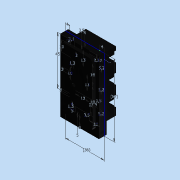
# Autodesk Inventor part: Base_V3
Saved by Autodesk Inventor 2015 (Build 190159000, 159)
## iProperties
Created: 2015-01-28
Part Number: Base_V3
Material: Generic
Document SubType Name: Modeling
Designer: Openlab
Density: 1 g/cm^3
Appearance: Smooth - Black
Author: Openlab
Autodesk Inventor part; units mm, degrees
ref_plane "YZ Plane" through (0, 0, 0) normal (1, 0, 0) x (0, 1, 0)
ref_plane "XZ Plane" through (0, 0, 0) normal (0, 1, 0) x (-1, 0, 0)
ref_plane "XY Plane" through (0, 0, 0) normal (0, 0, 1) x (1, 0, 0)
sketch "Sketch1" plane through (0, 0, 0) normal (0, 1, 0) x (-1, 0, 0)
  line L0 (23, -7.5) -> (10, -7.5)
  line L1 (10, -7.5) -> (10, -20.5)
  line L2 (10, -20.5) -> (23, -20.5)
  line L3 (10, -43.5) -> (10, -56.5)
  line L4 (10, -56.5) -> (23, -56.5)
  line L5 (23, -43.5) -> (10, -43.5)
  line L6 (0, -60) -> (0, 0)
  line L7 (28, -60) -> (0, -60)
  line L8 (23, -51.5) -> (28, -51.5)
  line L9 (28, -48.5) -> (23, -48.5)
  line L10 (24.85, -37) -> (26.15, -37)
  line L11 (26.15, -27) -> (24.85, -27)
  line L12 (28, -33.5) -> (26.15, -33.5)
  line L13 (24.85, -33.5) -> (23, -33.5)
  line L14 (28, -30.5) -> (26.15, -30.5)
  line L15 (24.85, -30.5) -> (23, -30.5)
  line L16 (23.95, -19) -> (27.05, -19)
  line L17 (27.05, -9) -> (23.95, -9)
  line L18 (23, -15.5) -> (23.95, -15.5)
  line L19 (27.05, -15.5) -> (28, -15.5)
  line L20 (23, -12.5) -> (23.95, -12.5)
  line L21 (27.05, -12.5) -> (28, -12.5)
  line L22 (0, -52.6) -> (10, -52.6)
  line L23 (0, -47.4) -> (10, -47.4)
  line L24 (0, -34.6) -> (10, -34.6)
  line L25 (0, -29.4) -> (10, -29.4)
  line L26 (0, -16.6) -> (10, -16.6)
  line L27 (0, -11.4) -> (10, -11.4)
  line L28 (30.1668, -14) -> (1.95, -14) construction
  line L29 (23, -7.5) -> (23, -20.5)
  line L30 (25.5, -5.5957) -> (25.5, -61.9523) construction
  line L31 (27.05, -9) -> (27.05, -19)
  line L32 (23.95, -9) -> (23.95, -19)
  line L33 (32.1467, -32) -> (-0.6768, -32) construction
  line L34 (26.15, -27) -> (26.15, -37)
  line L35 (24.85, -27) -> (24.85, -37)
  line L36 (1.6727, -50) -> (31.8542, -50) construction
  line L37 (28, 0) -> (28, -60)
  line L38 (23, -43.5) -> (23, -56.5)
  line L39 (23, -25.5) -> (10, -25.5)
  line L40 (10, -25.5) -> (10, -38.5)
  line L41 (10, -38.5) -> (23, -38.5)
  line L42 (23, -38.5) -> (23, -25.5)
  line L43 (16.5, -5.8794) -> (16.5, -56.7788) construction
  line L44 (28, 0) -> (0, 0)
  line L45 (28, 0) -> (32, 0)
  line L46 (32, 0) -> (32, -67)
  line L47 (32, -67) -> (-4, -67)
  line L48 (-4, -67) -> (-4, 0)
  line L49 (28, -5) -> (30, -5)
  line L50 (30, -5) -> (30, -50)
  line L51 (30, -50) -> (32, -50)
  line L52 (-4, 0) -> (0, 0)
  line L53 (0, -5) -> (-2, -5)
  line L54 (-2, -5) -> (-2, -65)
  line L55 (-2, -65) -> (32, -65)
  line L56 (28, -4) -> (0, -4)
  line L57 (38, -5) -> (-10, -5) construction
  line L58 (1.5, -47.4) -> (1.5, -43.4)
  line L59 (1.5, -43.4) -> (0, -43.4)
  line L60 (1.5, -29.4) -> (1.5, -25.4)
  line L61 (1.5, -25.4) -> (0, -25.4)
  line L62 (1.5, -11.4) -> (1.5, -7.4)
  line L63 (1.5, -7.4) -> (0, -7.4)
  line L64 (31, -55.75) -> (28.6955, -55.75) construction
  line L65 (28, -53.75) -> (26.5, -53.75)
  line L66 (26.5, -53.75) -> (26.5, -57.75)
  line L67 (26.5, -57.75) -> (28, -57.75)
  point P0 (16.5, -14)
  point P1 (16.5, -32)
  point P2 (16.5, -50)
  dimension "d0" = 13
  dimension "d7" = 1.3
  dimension "d8" = 10
  dimension "d9" = 3
  dimension "d10" = 3.1
  dimension "d11" = 10
  dimension "d12" = 5.2
  dimension "d13" = 5.2
  dimension "d14" = 5.2
  dimension "d15" = 10
  dimension "d17" = 13
  dimension "d18" = 18
  dimension "d19" = 18
  dimension "d20" = 13
  dimension "d21" = 5
  dimension "d23" = 3
  dimension "d24" = 13
  dimension "d26" = 3.5
  dimension "d36" = 4
  dimension "d38" = 2
  dimension "d39" = 45
  dimension "d40" = 4
  dimension "d41" = 2
  dimension "d44" = 3
  dimension "d59" = 3.5
  dimension "d63" = 5
  dimension "d64" = 2.5
  dimension "d65" = 2
  dimension "d66" = 4
  dimension "d67" = 67
  dimension "d68" = 36
  dimension "d95" = 4
  dimension "d96" = 1.5
  dimension "d99" = 4
  dimension "d100" = 1.5
  constraints: 132 end point, 37 point on line, 20 horizontal, 16 perpendicular, 12 collinear, 9 parallel, 8 vertical, 1 coincident, 43 other
  measures "d0" distance of L38.end L38.start
  measures "d7" distance of L35.start L34.start
  measures "d8" distance of L34.start L10.end
  measures "d9" distance between parallel lines of L14 L12
  measures "d10" distance of L32.start L31.start
  measures "d11" distance of L31.start L16.end
  measures "d12" distance between parallel lines of L27 L26
  measures "d13" distance between parallel lines of L25 L24
  measures "d14" distance between parallel lines of L22 L23
  measures "d15" distance of the line from the sketch origin of L3
  measures "d17" distance between parallel lines of L2 L0
  measures "d18" distance between parallel lines of L33 L28
  measures "d19" distance between parallel lines of L36 L33
  measures "d20" distance between parallel lines of L3 L38
  measures "d23" distance between parallel lines of L18 L20
  measures "d24" distance between parallel lines of L41 L39
  measures "d26" distance between parallel lines of L7 L4
  measures "d36" distance of L44.start L45.end
  measures "d38" distance of L49.start L49.end
  measures "d39" distance of L49.end L50.end
  measures "d40" distance of L48.end L44.end
  measures "d41" distance of L53.start L53.end
  measures "d44" distance between parallel lines of L8 L9
  measures "d59" distance between parallel lines of L56 L0
  measures "d63" distance between parallel lines of L55 L7
  measures "d64" distance between parallel lines of L0 L57
  measures "d65" distance between parallel lines of L47 L55
  measures "d66" distance between parallel lines of L44 L56
  measures "d67" distance of L47.end L48.end
  measures "d68" distance of L46.end L47.end
  measures "d95" distance of L58.start L58.end
  measures "d96" distance of L58.end L59.end
  measures "d99" distance of L65.end L66.end
  measures "d100" distance of L66.end L67.end
extrude "Extrusion2" add sketch "Sketch1" along normal blind 2.5 contours L53 L54 L55 L46 L47 L48 L52 L6 | L6 L44 L37 L56 | L37 L45 L46 L51 L50 L49
extrude "Extrusion3" add sketch "Sketch1" along normal blind 7.4 contours L20 L32 L18 L29 | L1 L26 L6 L27 | L21 L37 L19 L31 | L25 L40 L24 L6 | L37 L12 L34 L14 | L23 L3 L22 L6 | L37 L8 L38 L9 | L42 L15 L35 L13
extrude "Extrusion4" add sketch "Sketch1" against normal blind 4.8
sketch "Sketch2" plane through (0, -4.8, 0) normal (0, -1, 0) x (1, 0, 0)
  line L0 (-3, -3) -> (-25, -3)
  line L1 (-29, -7) -> (-29, -58)
  line L2 (-25, -62) -> (-3, -62)
  line L3 (1, -58) -> (1, -7)
  line L4 (4, -67) -> (4, 0) projected
  line L5 (4, 0) -> (-32, 0) projected
  line L6 (-32, 0) -> (-32, -67) projected
  line L7 (-32, -67) -> (4, -67) projected
  arc A0 (1, -7) -> (-3, -3) centre (-3, -7) ccw
  arc A1 (-3, -62) -> (1, -58) centre (-3, -58) ccw
  arc A2 (-29, -58) -> (-25, -62) centre (-25, -58) ccw
  arc A3 (-25, -3) -> (-29, -7) centre (-25, -7) ccw
  point P0 (0, 0)
  dimension "d53" = 3
  dimension "d54" = 3
  dimension "d55" = 3
  dimension "d56" = 5
  dimension "d85" = 8
  constraints: 8 end point, 8 point on circle, 8 tangent, 4 centre point, 2 horizontal alignment, 2 parallel, 1 horizontal, 1 perpendicular, 1 vertical alignment
  measures "d53" distance between parallel lines of L4 L3
  measures "d54" distance between parallel lines of L5 L0
  measures "d55" distance between parallel lines of L6 L1
  measures "d56" distance between parallel lines of L7 L2
  measures "d85" diameter of A0
extrude "Extrusion5" add sketch "Sketch2" along normal blind 3 contours A0 L3 A1 L2 A2 L1 A3 L0
extrude "Extrusion6" add sketch "Sketch1" along normal blind 15 contours L0 L1 L27 L62 L63 L6 L56 L37 L21 L31 L17 L32 L20 L29 | L18 L32 L16 L31 L19 L37 L14 L34 L11 L35 L15 L42 L39 L40 L25 L60 L61 L6 L26 L1 L2 L29 | L27 L6 L63 L62 | L61 L60 L25 L6 | L24 L40 L41 L42 L13 L35 L10 L34 L12 L37 L9 L38 L5 L3 L23 L58 L59 L6 | L59 L58 L23 L6 | L22 L3 L4 L38 L8 L37 L65 L66 L67 L7 L6 | L37 L67 L66 L65
sketch "Sketch3" plane through (0, 0, -5) normal (1, 0, 0) x (0, 0, -1)
  circle A0 centre (9, 10) radius 3.1
  line L0 (60, 0) -> (0, 0) projected
  line L1 (5.9, 10) -> (5.9, 15)
  line L2 (5.9, 15) -> (12.1, 15)
  line L3 (12.1, 15) -> (12.1, 10)
  line L4 (-5, -4.8) -> (-5, 2.5) projected
  circle A1 centre (27, 10) radius 3.1
  line L5 (23.9, 10) -> (23.9, 15)
  line L6 (23.9, 15) -> (30.1, 15)
  line L7 (30.1, 15) -> (30.1, 10)
  circle A2 centre (45, 10) radius 3.1
  line L8 (41.9, 10) -> (41.9, 15)
  line L9 (41.9, 15) -> (48.1, 15)
  line L10 (48.1, 15) -> (48.1, 10)
  point P0 (-5, 0)
  point P1 (0, 2.5)
  dimension "d69" = 6.2
  dimension "d70" = 10
  dimension "d72" = 9
  dimension "d74" = 5
  dimension "d75" = 6.2
  dimension "d76" = 18
  dimension "d77" = 5
  dimension "d78" = 6.2
  dimension "d79" = 18
  dimension "d80" = 5
  constraints: 18 end point, 6 perpendicular, 6 point on circle, 6 tangent, 3 centre point, 2 horizontal alignment, 2 vertical, 1 horizontal
  measures "d69" diameter of A0
  measures "d70" distance from line of L0 A0.centre
  measures "d72" horizontal distance of point (0, 2.5) A0.centre
  measures "d74" distance from line of L2 A0.centre
  measures "d75" diameter of A1
  measures "d76" distance of A1.centre A0.centre
  measures "d77" distance from line of L6 A1.centre
  measures "d78" diameter of A2
  measures "d79" distance of A2.centre A1.centre
  measures "d80" distance from line of A2.centre L9
extrude "Extrusion7" cut sketch "Sketch3" against normal blind 1.5
fillet "Fillet1" radius 2.5 6 edges at (-5, 7.4, -29.4) (-5, 7.4, -34.6) (-5, 7.4, -47.4) (-5, 7.4, -52.6) (-5, 7.4, -16.6) (-5, 7.4, -11.4)
hole "Hole1" at (-16.5, 0, -14) at (-16.5, 0, -32) at (-16.5, 0, -50) direction (0, -1, 0) diameter 3 end through all countersink diameter 8 countersink angle 90
extrude "Extrusion8" cut sketch "Sketch1" against normal blind 0.5 contours L6 L7 L37 L49 L50 L51 L46 L55 L54 L53
extrude "Extrusion9" cut sketch "Sketch1" along normal up to next contours L27 L6 L63 L62 | L61 L60 L25 L6 | L59 L58 L23 L6 | L37 L67 L66 L65
body "Solid1"
